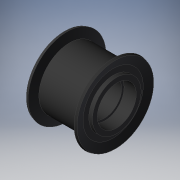
# Autodesk Inventor part: C-AFDF22-25_bw
Saved by Autodesk Inventor 2019 (Build 230136000, 136)
## iProperties
Created: 2023-11-09
Part Number: C-AFDF22-25_bw
Material: Generic
Catalog Web Link: www.cadenas.de
Description: C-AFBD-W, C-AFDF-W_bw-Economy Idlers Backside Tension Type
Vendor: MISUMI
Document SubType Name: Modeling
Designer: psAdmin
Manufacturer: MISUMI
Mass: 7.03363 g
Surface Area: 46.7242 cm^2
Volume: 7.03363 cm^3
Density: 1 g/cm^3
Appearance: PSOLRGB-175-175-175
Category: PARTsolutions
Company: MISUMI
Title: C-AFDF22-25
Author: Cadenas PARTsolutions
Comments: Economy Idlers Backside Tension Type
PSOL_IDENT_0: {$CADENAS_DATA/23d-libs/misumi/metric/51_timing_pulleys/c_afbd/c_afbd_w_body.prj},183 {VTYP=3D},{NB=
PSOL_IDENT_1: C-AFDF22-25_bw},{LINA=C-AFDF22-25},{NN=C-AFBD-W, C-AFDF-W_bw},{DATE=13.09.2022 06:55:24},{GEOMDATE=1
PSOL_IDENT_2: 8.05.2021 06:11:19},{VERSION=},{LINEID=100},{WBVAR=TS},{WBNUMERIC=}  {NB=C-AFDF22-25_bw},{LINA=C-AFD
PSOL_IDENT_3: F22-25},{KT=DUMMY},{PN=C-AFDF22-25},{TYPE=C-AFDF},{TS=C-AFDF},{TSALG= 'C-AFBD','No Flange','C-AFDF','
PSOL_IDENT_4: Flanged' },{W=22},{NOM=25},{NOMALG= '25','35W' },{D=25},{F=32},{A=17},{ABI=-},{ABM=150},{NO=688ZZ×2}
PSOL_IDENT_5: ,{BN=688},{DD=8},{B=5.0},{E=20.000},{BD=16.000},{DH=14.000},{PTT=1.000},{CIF=1.000}
NB: C-AFDF22-25_bw
NN: C-AFBD-W, C-AFDF-W_bw
NT: Economy Idlers Backside Tension Type
NBSYN: $PN._bw
LINA: C-AFDF22-25
CATALOG: Misumi
PN: C-AFDF22-25
TYPE: C-AFDF
TS: Flanged
W: 22
NOM: 25
D: 25
F: 32
A: 17
ABI: -
ABM: 150
NO: 688ZZ×2
BN: 688
DD: 8
B: 5
SUPPLIER: MISUMI
ARTICLENO: C-AFDF22-25_bw
BOMINFO: C-AFDF22-25
CREATOR: CADENAS GmbH
Autodesk Inventor part; units mm, degrees
sketch "_____2" plane through (0, 0, 0) normal (0, 0, 1) x (1, 0, 0)
  line L0 (11, 0) -> (-11, 0)
  line L1 (-11, 0) -> (-11, 10)
  line L2 (-11, 10) -> (-9.5, 10)
  line L3 (-9.5, 10) -> (-9.5, 12.3683)
  line L4 (-9.5, 12.3683) -> (-10.4037, 15.7412)
  line L5 (-10.4037, 15.7412) -> (-9.4378, 16)
  line L6 (-9.4378, 16) -> (-8.5, 12.5)
  line L7 (-8.5, 12.5) -> (8.5, 12.5)
  line L8 (8.5, 12.5) -> (9.4378, 16)
  line L9 (9.4378, 16) -> (10.4037, 15.7412)
  line L10 (10.4037, 15.7412) -> (9.5, 12.3683)
  line L11 (9.5, 12.3683) -> (9.5, 10)
  line L12 (9.5, 10) -> (11, 10)
  line L13 (11, 10) -> (11, 0)
  line L14 (11, 0) -> (-11, 0)
  constraints: 30 end point
revolve "Revolution1" add sketch "_____2" angle 360 about axis through (11, 0, 0) along (1, 0, 0)
sketch "_____3" plane through (0, 0, 0) normal (0, 0, 1) x (1, 0, 0)
  line L0 (11, 0) -> (-11, 0)
  line L1 (-11, 0) -> (-11, 8)
  line L2 (-11, 8) -> (-6, 8)
  line L3 (-6, 8) -> (-6, 7)
  line L4 (-6, 7) -> (6, 7)
  line L5 (6, 7) -> (6, 8)
  line L6 (6, 8) -> (11, 8)
  line L7 (11, 8) -> (11, 0)
  line L8 (11, 0) -> (-11, 0)
  constraints: 18 end point
revolve "Revolution2" cut sketch "_____3" angle 360 about axis through (11, 0, 0) along (1, 0, 0)
ref_plane "b600_1_XY" through (8.5, 0, 0) normal (1, 0, 0) x (0, 0, -1)
ref_plane "b600_1_YZ" through (8.5, 0, 0) normal (0, 0, -1) x (0, 1, 0)
ref_plane "b600_1_ZX" through (8.5, 0, 0) normal (0, 1, 0) x (1, 0, 0)
ref_plane "b600_2_XY" through (-8.5, 0, 0) normal (1, 0, 0) x (0, 0, -1)
ref_plane "b600_2_YZ" through (-8.5, 0, 0) normal (0, 0, -1) x (0, 1, 0)
ref_plane "b600_2_ZX" through (-8.5, 0, 0) normal (0, 1, 0) x (1, 0, 0)
ref_plane "to_dummy_XY" through (0, 0, 0) normal (1, 0, 0) x (0, 0, -1)
ref_plane "to_dummy_YZ" through (0, 0, 0) normal (0, 0, -1) x (0, 1, 0)
ref_plane "to_dummy_ZX" through (0, 0, 0) normal (0, 1, 0) x (1, 0, 0)
body "Solid1"
